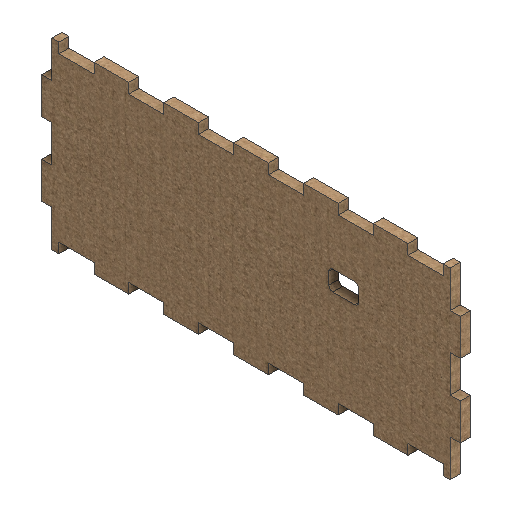
# Autodesk Inventor part: Backplate
Saved by Autodesk Inventor 2025.2 (Build 292293000, 293)
## iProperties
Created: 2025-03-07
Part Number: Backplate
Material: MDF Medium Density Fiberboard
Document SubType Name: Modeling
Designer: ahorat
Density: 0.8 g/cm^3
Appearance: Cardboard - Corrugated
Author: ahorat
Autodesk Inventor part; units mm, degrees
ref_plane "YZ Plane" through (0, 0, 0) normal (1, 0, 0) x (0, 1, 0)
ref_plane "XZ Plane" through (0, 0, 0) normal (0, 1, 0) x (-1, 0, 0)
ref_plane "XY Plane" through (0, 0, 0) normal (0, 0, 1) x (1, 0, 0)
sketch "Sketch1" plane through (0, 0, 0) normal (0, 0, 1) x (1, 0, 0)
  line L0 (-105, -46) -> (105, -46)
  line L1 (105, -46) -> (105, 46)
  line L2 (105, 46) -> (-105, 46)
  line L3 (-105, 46) -> (-105, -46)
  line L4 (-105, -46) -> (105, 46) construction
  line L5 (105, -46) -> (-105, 46) construction
  point P0 (0, 0)
  dimension "d0" = 210
  dimension "d1" = 92
  constraints: 12 end point, 2 midpoint, 2 parallel, 1 horizontal, 1 perpendicular
  measures "d0" distance of L1.end L2.end
  measures "d1" distance of L0.end L1.end
extrude "Extrusion1" add sketch "Sketch1" along normal blind 5
sketch "Sketch2" plane through (0, 0, 5) normal (0, 0, 1) x (1, 0, 0)
  line L0 (39, 16.1) -> (54, 16.1)
  line L1 (54, 16.1) -> (54, 6.1)
  line L2 (54, 6.1) -> (39, 6.1)
  line L3 (39, 6.1) -> (39, 16.1)
  line L4 (-3, 9.6) -> (85, 9.6) construction
  line L5 (85, 9.6) -> (85, 8) construction
  line L6 (85, 8) -> (-3, 8) construction
  line L7 (-3, 8) -> (-3, 9.6) construction
  line L8 (-105, -46) -> (105, -46) construction
  line L9 (7.25, 15.6) -> (17.25, 15.6)
  line L10 (17.25, 15.6) -> (17.25, 10.6)
  line L11 (17.25, 10.6) -> (7.25, 10.6)
  line L12 (7.25, 10.6) -> (7.25, 15.6)
  line L13 (105, -46) -> (105, 46) projected
  line L14 (17.25, 10.6) -> (7.25, 15.6) construction
  line L15 (17.25, 15.6) -> (7.25, 10.6) construction
  line L16 (54, 6.1) -> (39, 16.1) construction
  line L17 (39, 6.1) -> (54, 16.1) construction
  point P0 (0, 0)
  point P1 (85, 8.8)
  point P2 (54, 11.1)
  point P3 (12.25, 13.1)
  point P4 (12.25, 13.1)
  point P5 (46.5, 11.1)
  point P6 (46.5, 11.1)
  dimension "d4" = 1.6
  dimension "d5" = 55.6
  dimension "d7" = 15
  dimension "d8" = 10
  dimension "d9" = 10
  dimension "d10" = 5
  dimension "d12" = 88
  dimension "d13" = 20
  dimension "d17" = 3.5
  dimension "d18" = 72.75
  dimension "d19" = 1.5
  dimension "d20" = 38.5
  constraints: 32 end point, 6 midpoint, 6 parallel, 3 horizontal, 3 perpendicular
  measures "d4" distance of L6.end L4.start
  measures "d5" distance between parallel lines of L8 L4
  measures "d7" distance of L0.start L0.end
  measures "d8" distance between parallel lines of L2 L0
  measures "d9" distance of L9.start L9.end
  measures "d10" distance of L11.end L9.start
  measures "d12" distance of L5.end L6.end
  measures "d13" distance from line of L13 point (85, 8.8)
  measures "d17" distance from line of point (12.25, 13.1) L4
  measures "d18" horizontal distance of point (85, 8.8) point (12.25, 13.1)
  measures "d19" distance from line of L4 point (46.5, 11.1)
  measures "d20" horizontal distance of point (85, 8.8) point (46.5, 11.1)
extrude "Extrusion2" cut sketch "Sketch2" against normal blind 5 contours L0 L1 L2 L3
fillet "Fillet1" radius 2 4 edges at (39, 16.1, 2.5) (39, 6.1, 2.5) (54, 6.1, 2.5) (54, 16.1, 2.5)
sketch "Sketch3" plane through (0, 0, 5) normal (0, 0, 1) x (1, 0, 0)
  line L0 (-8.75, 46) -> (-26.35, 46)
  line L1 (-26.35, 46) -> (-26.35, 40.9)
  line L2 (-26.35, 40.9) -> (-8.75, 40.9)
  line L3 (-8.75, 40.9) -> (-8.75, 46)
  line L4 (-43.75, 46) -> (-61.35, 46)
  line L5 (-61.35, 46) -> (-61.35, 40.9)
  line L6 (-61.35, 40.9) -> (-43.75, 40.9)
  line L7 (-43.75, 40.9) -> (-43.75, 46)
  line L8 (-78.75, 46) -> (-96.35, 46)
  line L9 (-96.35, 46) -> (-96.35, 40.9)
  line L10 (-96.35, 40.9) -> (-78.75, 40.9)
  line L11 (-78.75, 40.9) -> (-78.75, 46)
  line L12 (0, 0) -> (0, 46) construction
  line L13 (78.75, 40.9) -> (78.75, 46)
  line L14 (96.35, 40.9) -> (78.75, 40.9)
  line L15 (96.35, 46) -> (96.35, 40.9)
  line L16 (78.75, 46) -> (96.35, 46)
  line L17 (8.75, 40.9) -> (8.75, 46)
  line L18 (26.35, 40.9) -> (8.75, 40.9)
  line L19 (8.75, 46) -> (26.35, 46)
  line L20 (26.35, 46) -> (26.35, 40.9)
  line L21 (43.75, 40.9) -> (43.75, 46)
  line L22 (61.35, 46) -> (61.35, 40.9)
  line L23 (43.75, 46) -> (61.35, 46)
  line L24 (61.35, 40.9) -> (43.75, 40.9)
  line L25 (0, 0) -> (105, 0) construction
  line L26 (-96.35, -40.9) -> (-78.75, -40.9)
  line L27 (-78.75, -40.9) -> (-78.75, -46)
  line L28 (-78.75, -46) -> (-96.35, -46)
  line L29 (-61.35, -40.9) -> (-43.75, -40.9)
  line L30 (-43.75, -40.9) -> (-43.75, -46)
  line L31 (-43.75, -46) -> (-61.35, -46)
  line L32 (-26.35, -46) -> (-26.35, -40.9)
  line L33 (-26.35, -40.9) -> (-8.75, -40.9)
  line L34 (-96.35, -46) -> (-96.35, -40.9)
  line L35 (-61.35, -46) -> (-61.35, -40.9)
  line L36 (-8.75, -40.9) -> (-8.75, -46)
  line L37 (-8.75, -46) -> (-26.35, -46)
  line L38 (8.75, -40.9) -> (8.75, -46)
  line L39 (26.35, -40.9) -> (8.75, -40.9)
  line L40 (8.75, -46) -> (26.35, -46)
  line L41 (26.35, -46) -> (26.35, -40.9)
  line L42 (43.75, -40.9) -> (43.75, -46)
  line L43 (61.35, -46) -> (61.35, -40.9)
  line L44 (43.75, -46) -> (61.35, -46)
  line L45 (61.35, -40.9) -> (43.75, -40.9)
  line L46 (78.75, -40.9) -> (78.75, -46)
  line L47 (78.75, -46) -> (96.35, -46)
  line L48 (96.35, -46) -> (96.35, -40.9)
  line L49 (96.35, -40.9) -> (78.75, -40.9)
  line L50 (105, 46) -> (-105, 46) projected
  line L51 (-105, 46) -> (-105, -46) projected
  line L52 (-105, -46) -> (105, -46) projected
  line L53 (105, -46) -> (105, 46) projected
  line L54 (-105, 46) -> (-99.9, 46)
  line L55 (-99.9, 46) -> (-99.9, 27.5)
  line L56 (-99.9, 27.5) -> (-105, 27.5)
  line L57 (-105, 27.5) -> (-105, 46)
  line L58 (-105, -46) -> (-99.9, -46)
  line L59 (-99.9, -46) -> (-99.9, -27.5)
  line L60 (-99.9, -27.5) -> (-105, -27.5)
  line L61 (-105, -27.5) -> (-105, -46)
  line L62 (-105, -9.25) -> (-99.9, -9.25)
  line L63 (-99.9, -9.25) -> (-99.9, 9.25)
  line L64 (-99.9, 9.25) -> (-105, 9.25)
  line L65 (-105, 9.25) -> (-105, -9.25)
  line L66 (105, 46) -> (99.9, 46)
  line L67 (99.9, 46) -> (99.9, 27.5)
  line L68 (99.9, 27.5) -> (105, 27.5)
  line L69 (105, 27.5) -> (105, 46)
  line L70 (105, -46) -> (99.9, -46)
  line L71 (99.9, -46) -> (99.9, -27.5)
  line L72 (99.9, -27.5) -> (105, -27.5)
  line L73 (105, -27.5) -> (105, -46)
  line L74 (105, -9.25) -> (99.9, -9.25)
  line L75 (99.9, -9.25) -> (99.9, 9.25)
  line L76 (99.9, 9.25) -> (105, 9.25)
  line L77 (105, 9.25) -> (105, -9.25)
  point P0 (-17.55, 40.9)
  point P1 (-52.55, 40.9)
  point P2 (-87.55, 40.9)
  point P3 (87.55, 40.9)
  point P4 (17.55, 40.9)
  point P5 (52.55, 40.9)
  point P6 (-87.55, -40.9)
  point P7 (-52.55, -40.9)
  point P8 (-17.55, -40.9)
  point P9 (0, -46)
  point P10 (17.55, -40.9)
  point P11 (52.55, -40.9)
  point P12 (87.55, -40.9)
  point P13 (-105, 0)
  dimension "d27" = 17.55
  dimension "d28" = 17.6
  dimension "d29" = 5.1
  dimension "d30" = 35
  dimension "d32" = 210
  dimension "d35" = 92
  dimension "d38" = 18.5
  constraints: 148 end point, 56 symmetric about line, 8 parallel, 6 point on line, 5 horizontal, 5 midpoint, 4 perpendicular, 3 equal length, 1 coincident, 1 vertical, 18 other
  measures "d27" horizontal distance of L12.end point (-17.55, 40.9)
  measures "d28" distance of L1.end L2.end
  measures "d29" distance of L0.end L1.end
  measures "d30" distance of L0.start L4.start
  measures "d32" distance of L50.start L50.end
  measures "d35" distance of L50.end L51.end
  measures "d38" distance of L64.end L62.start
extrude "Extrusion3" cut sketch "Sketch3" against normal blind 5 contours L3 L2 L1 L0 | L19 L20 L18 L17 | L7 L6 L5 L4 | L23 L22 L24 L21 | L11 L10 L9 L8 | L16 L15 L14 L13 | L55 L56 L51 L50 | L50 L53 L68 L67 | L64 L63 L62 L51 | L53 L74 L75 L76 | L60 L59 L52 L51 | L53 L52 L71 L72 | L34 L26 L27 L28 | L47 L46 L49 L48 | L35 L29 L30 L31 | L44 L42 L45 L43 | L32 L33 L36 L37 | L40 L38 L39 L41
equation "\"d30\" = 0.166667 * d32"
body "Solid1"
